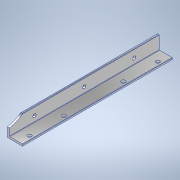
# Autodesk Inventor part: 1in Angle x 250
Saved by Autodesk Inventor 2022 (Build 260153000, 153)
## iProperties
Created: 2022-10-12
Part Number: 1in Angle x 250
Material: Aluminum 6061
Document SubType Name: Modeling
Designer: matt
Density: 2.7 g/cm^3
Appearance: Aluminum - Flat
Mass: 105.216 g
Surface Area: 252.898 cm^2
Volume: 38.9688 cm^3
Author: matt
Autodesk Inventor part; units mm, degrees
ref_plane "YZ Plane" through (0, 0, 0) normal (1, 0, 0) x (0, 1, 0)
ref_plane "XZ Plane" through (0, 0, 0) normal (0, 1, 0) x (-1, 0, 0)
ref_plane "XY Plane" through (0, 0, 0) normal (0, 0, 1) x (1, 0, 0)
sketch "Sketch1" plane through (0, 0, 0) normal (0, 0, 1) x (1, 0, 0)
  line L0 (0.5, 0) -> (3.3, 0)
  line L1 (3.3, 3.8) -> (3.3, 24.8)
  line L2 (2.8, 25.3) -> (0.5, 25.3)
  line L3 (0, 24.8) -> (0, 0.5)
  line L4 (0, 0) -> (24.8, 0)
  line L5 (25.3, 0.5) -> (25.3, 2.8)
  line L6 (24.8, 3.3) -> (3.8, 3.3)
  line L7 (0, 3.3) -> (0, 0)
  arc A0 (3.3, 24.8) -> (2.8, 25.3) centre (2.8, 24.8) ccw
  arc A1 (0.5, 25.3) -> (0, 24.8) centre (0.5, 24.8) ccw
  arc A2 (3.3, 3.8) -> (3.8, 3.3) centre (3.8, 3.8) ccw
  arc A3 (0, 0.5) -> (0.5, 0) centre (0.5, 0.5) ccw
  arc A4 (24.8, 0) -> (25.3, 0.5) centre (24.8, 0.5) ccw
  arc A5 (25.3, 2.8) -> (24.8, 3.3) centre (24.8, 2.8) ccw
  point P0 (3.3, 25.3)
  point P1 (0, 25.3)
  point P2 (25.3, 3.3)
  point P3 (25.3, 0)
  dimension "d0" = 3.3
  dimension "d1" = 25.3
  dimension "d2" = 25.3
  dimension "d3" = 3.3
  dimension "d4" = 0.5
  constraints: 16 end point, 12 point on circle, 12 tangent, 10 point on line, 6 centre point, 5 equal radius, 4 parallel, 2 horizontal, 2 perpendicular
  measures "d0" distance of point (0, 25.3) point (3.3, 25.3)
  measures "d1" distance of point (3.3, 25.3) L0.end
  measures "d2" distance of L7.start point (25.3, 3.3)
  measures "d3" distance of point (25.3, 3.3) point (25.3, 0)
  measures "d4" radius of A0
extrude "Extrusion1" add sketch "Sketch1" along normal blind 249.043 contours A3 L3 A1 L2 A0 L1 A2 L6 A5 L5 A4 L4 L0
sketch "Sketch2" plane through (3.8, 3.3, 0) normal (0, 1, 0) x (1, 0, 0)
  circle A0 centre (15, -231.1777) radius 3.3
  line L0 (21, -249.043) -> (0, -249.043) projected
  line L1 (-3.8, 0) -> (-3.8, -249.043) construction
  line L2 (-3.8, -124.5215) -> (21, -124.5215) construction
  line L3 (21, 0) -> (21, -249.043) construction
  circle A1 centre (15, -17.8653) radius 3.3
  line L4 (15, -231.1777) -> (15, -124.5215) construction
  line L5 (15, -124.5215) -> (15, -17.8653) construction
  circle A2 centre (15, -75.1918) radius 3.3
  circle A3 centre (15, -173.8512) radius 3.3
  dimension "d7" = 6.6
  dimension "d9" = 6
  dimension "d12" = 213.3123
  dimension "d23" = 6.6
  constraints: 6 end point, 4 centre point, 2 collinear, 2 midpoint, 1 perpendicular, 1 point on line, 1 symmetric about line, 1 other
  measures "d7" diameter of A0
  measures "d9" distance from line of L3 L4.start
  measures "d12" distance of L5.end L4.start
  measures "d23" diameter of A2
extrude "Extrusion2" cut sketch "Sketch2" against normal through all
sketch "Sketch3" plane through (3.3, 3.8, 0) normal (1, 0, 0) x (0, 0, -1)
  line L0 (-249.043, 21) -> (-249.043, -3.3) construction
  line L1 (-249.043, 8.85) -> (0, 8.85) construction
  line L2 (0, 21) -> (0, -3.3) projected
  circle A0 centre (-124.5215, 8.85) radius 2.8
  circle A1 centre (-207.5358, 8.85) radius 2.8
  circle A2 centre (-41.5072, 8.85) radius 2.8
  line L3 (-249.043, 0) -> (-249.043, 21) projected
  line L4 (0, 21.5) -> (-249.043, 21.5) projected
  line L5 (-249.043, 21.5) -> (-249.043, 21) projected
  arc A3 (-262.8543, 11.011) -> (-243.3985, 118.5449) centre (-259.3098, 65.8967) ccw projected
  point P0 (0, -3.8)
  point P1 (-249.043, 11.8634)
  point P2 (-226.8454, 21.5)
  dimension "d14" = 5.6
  dimension "d15" = 249.043
  dimension "d16" = 124.5215
  dimension "d17" = 5.6
  dimension "d18" = 5.6
  dimension "d19" = 41.5072
  dimension "d20" = 41.5072
  constraints: 3 centre point, 3 midpoint, 2 end point, 2 point on line
  measures "d14" diameter of A0
  measures "d15" distance between parallel lines of L2 L0
  measures "d16" distance from line of L0 A0.centre
  measures "d17" diameter of A1
  measures "d18" diameter of A2
  measures "d19" distance from line of L2 A2.centre
  measures "d20" distance from line of A1.centre L0
extrude "Extrusion3" cut sketch "Sketch3" against normal blind 10
equation "\"d16\" = 0.5 * d15"
equation "\"d19\" = 0.333333 * d16"
equation "\"d20\" = 0.333333 * d16"
body "Solid1"
